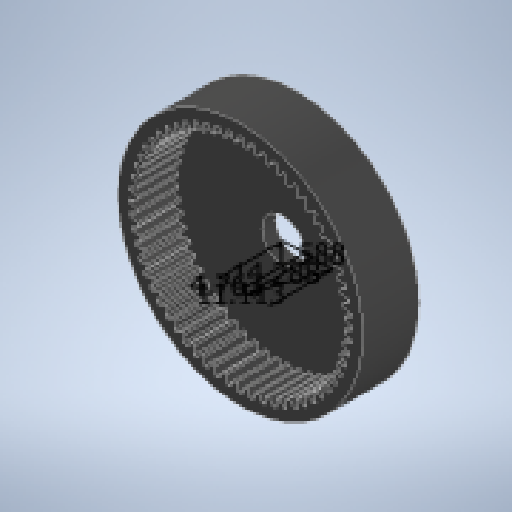
# Autodesk Inventor part: Spur Gear2
Saved by Autodesk Inventor 2023.2 (Build 272271000, 271)
## iProperties
CustomPartVersion: 1
Created: 2023-02-28
Part Number: Spur Gear2
Material: Nylon 6/6
Document SubType Name: Modeling
Designer: Nathan Cai
Categories: <?xml version="1.0" encoding="UTF-16"?> <MemberInstance><Categories><FamilyTemplate><FamilyTemplateParameter ValueType="xs:double" Id="1" ObjectReferenceKey="da_z" ObjectType="kUserParameterObject"/><FamilyTemplateParameter ValueType="xs:double" Id="2" ObjectReferenceKey="da_b" ObjectType="kUserParameterObject"/><FamilyTemplateParameter ValueType="xs:double" Id="3" ObjectReferenceKey="da_beta" ObjectType="kUserParameterObject"/><FamilyTemplateParameter ValueType="xs:double" Id="4" ObjectReferenceKey="da_da" ObjectType="kUserParameterObject"/><FamilyTemplateParameter ValueType="xs:double" Id="5" ObjectReferenceKey="da_aw" ObjectType="kUserParameterObject"/><FamilyTemplateParameter ValueType="xs:string" Id="6" ObjectReferenceKey="EAIAABAAAACIAQAAAAAAAIAAAAAAAAAA" ObjectType="83910656" SubObjectId="SurfaceGeometry"/></FamilyTemplate><ParamToTemplateMap><ParamToTemplate CategoryParameter="//CategoryParameter[@InternalName='046C89C9-8512-4d59-83FE-43B91F4F132A']" TemplateParameter="1"/><ParamToTemplate CategoryParameter="//CategoryParameter[@InternalName='2552DF32-E462-4b46-AEBF-C6C7768E72AC']" TemplateParameter="2"/><ParamToTemplate CategoryParameter="//CategoryParameter[@InternalName='C9EE641D-15FC-4fae-A226-E94C4372FDD7']" TemplateParameter="3"/><ParamToTemplate><ParamToTemplate CategoryParameter="//CategoryParameter[@InternalName='00B6519A-459B-49c7-AD84-2E56D39A5744']" ConstantValue="-0.000000"/></ParamToTemplate><ParamToTemplate><ParamToTemplate CategoryParameter="//CategoryParameter[@InternalName='04B31F0E-C7A6-4894-AA32-9629BEFACF47']" ConstantValue="1.000000"/></ParamToTemplate><ParamToTemplate><ParamToTemplate CategoryParameter="//CategoryParameter[@InternalName='43CBEC2E-7847-49e7-A936-2F7889FCB2D9']" ConstantValue="0.250000"/></ParamToTemplate><ParamToTemplate><ParamToTemplate CategoryParameter="//CategoryParameter[@InternalName='B1EFC894-105D-4ebd-86BF-FA20ED196853']" ConstantValue="0.350000"/></ParamToTemplate><ParamToTemplate><ParamToTemplate CategoryParameter="//CategoryParameter[@InternalName='51175063-3D10-4879-93E8-6246FE8B403D']" ConstantValue="2060000000.000000"/></ParamToTemplate><ParamToTemplate><ParamToTemplate CategoryParameter="//CategoryParameter[@InternalName='A3A52E27-4454-46a9-B0BD-C932399B70AF']" ConstantValue="0.300000"/></ParamToTemplate><ParamToTemplate><ParamToTemplate CategoryParameter="//CategoryParameter[@InternalName='91B76062-C214-41d9-B1B9-14D2AB99603D']" ConstantValue="0.080000"/></ParamToTemplate><ParamToTemplate><ParamToTemplate CategoryParameter="//CategoryParameter[@InternalName='374E806E-8B8A-4dda-A9AA-1039D6500AD2']" ConstantValue="12.500000"/></ParamToTemplate><ParamToTemplate><ParamToTemplate CategoryParameter="//CategoryParameter[@InternalName='2D373A89-B862-43d6-8D0B-0CBF12AB9F6C']" ConstantValue="0.349066"/></ParamToTemplate><ParamToTemplate CategoryParameter="//CategoryParameter[@InternalName='37777632-D6A2-4fac-9D53-DB8ACD95C989']" TemplateParameter="4"/><ParamToTemplate CategoryParameter="//CategoryParameter[@InternalName='FD1017F1-B727-4f7e-9707-0F86F1FF9423']" TemplateParameter="5"/><ParamToTemplate><ParamToTemplate CategoryParameter="//CategoryParameter[@InternalName='9E1B4470-B2D3-4ff1-B813-535BB4CDF51A']" ConstantValue="3520000.000000"/></ParamToTemplate><ParamToTemplate><ParamToTemplate CategoryParameter="//CategoryParameter[@InternalName='F8452263-BFF6-458c-9FB1-07C4B99E95CD']" ConstantValue="11400000.000000"/></ParamToTemplate><ParamToTemplate><ParamToTemplate CategoryParameter="//CategoryParameter[@InternalName='3E3BB259-FD49-497f-8171-6EBC954A3479']" ConstantValue="2.000000"/></ParamToTemplate><ParamToTemplate CategoryParameter="//CategoryParameter[@InternalName='27C3BAF2-7550-4e4b-AE2C-0DB134B7D9B7']" TemplateParameter="6"/></ParamToTemplateMap><Category DisplayName="Gear" InternalName="DC85795E-93AB-48d5-8EEE-5A27447B64BD" Mnemonic="Gear"><CategoryParameter DisplayName="z" InternalName="046C89C9-8512-4d59-83FE-43B91F4F132A" Mnemonic="z"/><CategoryParameter DisplayName="b" InternalName="2552DF32-E462-4b46-AEBF-C6C7768E72AC" Mnemonic="b"/><CategoryParameter DisplayName="||b|" InternalName="C9EE641D-15FC-4fae-A226-E94C4372FDD7" Mnemonic="beta"/><CategoryParameter DisplayName="x" InternalName="00B6519A-459B-49c7-AD84-2E56D39A5744" Mnemonic="x"/><CategoryParameter DisplayName="a*" InternalName="04B31F0E-C7A6-4894-AA32-9629BEFACF47" Mnemonic="a"/><CategoryParameter DisplayName="c*" InternalName="43CBEC2E-7847-49e7-A936-2F7889FCB2D9" Mnemonic="c"/><CategoryParameter DisplayName="r|.f|*" InternalName="B1EFC894-105D-4ebd-86BF-FA20ED196853" Mnemonic="rf"/><CategoryParameter DisplayName="E" InternalName="51175063-3D10-4879-93E8-6246FE8B403D" Mnemonic="E"/><CategoryParameter DisplayName="||m|" InternalName="A3A52E27-4454-46a9-B0BD-C932399B70AF" Mnemonic="mi"/><Category DisplayName="SpurGear" InternalName="26C5A22E-A91E-4dfd-A3B3-23CCAFAE1764" Mnemonic="SpurGear"><CategoryParameter DisplayName="m" InternalName="91B76062-C214-41d9-B1B9-14D2AB99603D" Mnemonic="m"/><CategoryParameter DisplayName="P" InternalName="374E806E-8B8A-4dda-A9AA-1039D6500AD2" Mnemonic="PP"/><CategoryParameter DisplayName="||a|" InternalName="2D373A89-B862-43d6-8D0B-0CBF12AB9F6C" Mnemonic="alpha"/><CategoryParameter DisplayName="d|.a|" InternalName="37777632-D6A2-4fac-9D53-DB8ACD95C989" Mnemonic="da"/><CategoryParameter DisplayName="a|.w|" InternalName="FD1017F1-B727-4f7e-9707-0F86F1FF9423" Mnemonic="aw"/><CategoryParameter DisplayName="||s||.Flim|" InternalName="9E1B4470-B2D3-4ff1-B813-535BB4CDF51A" Mnemonic="sFlim"/><CategoryParameter DisplayName="||s||.Hlim|" InternalName="F8452263-BFF6-458c-9FB1-07C4B99E95CD" Mnemonic="sHlim"/><CategoryParameter DisplayName="type" InternalName="3E3BB259-FD49-497f-8171-6EBC954A3479" Mnemonic="type"/><Category DisplayName="InternalSpurGear" InternalName="7CF704F6-14A9-42f8-93CE-E71DF57C2B55" Mnemonic="InternalSpurGear"><CategoryParameter DisplayName="PitchDiameter" InternalName="27C3BAF2-7550-4e4b-AE2C-0DB134B7D9B7" Mnemonic="IDS_PITCHDIAM"/></Category></Category></Category></Categories></MemberInstance>
Density: 1.13 g/cm^3
Appearance: Rubber - Black
Mass: 12.9636 g
Surface Area: 87.0105 cm^2
Volume: 11.4722 cm^3
Author: Nathan Cai
Autodesk Inventor part; units mm, degrees
ref_plane "YZ Plane" through (0, 0, 0) normal (1, 0, 0) x (0, 1, 0)
ref_plane "XZ Plane" through (0, 0, 0) normal (0, 1, 0) x (-1, 0, 0)
ref_plane "XY Plane" through (0, 0, 0) normal (0, 0, 1) x (1, 0, 0)
sketch "Sketch1" plane through (0, 0, 0) normal (0, 0, 1) x (1, 0, 0)
  circle A0 centre (0, 0) radius 27.5
  dimension "d0" = 55
  constraints: 1 centre point
  measures "d0" diameter of A0
extrude "Extrusion1" add sketch "Sketch1" along normal blind 9.525
spur gear teeth "Spur Gear" teeth 60 pitch diameter 48 tip diameter 46.7556 root diameter 50 face width 9.525 start plane through (0, 0, 0) normal (0, 0, -1) x (-1, 0, 0)
sketch "Sketch4" plane through (0, 0, 0) normal (0, 0, -1) x (-1, 0, 0)
  circle A0 centre (0, 0) radius 27.5
  circle A1 centre (0, 0) radius 4.7625
  dimension "d55" = 55
  dimension "d56" = 9.525
  constraints: 2 centre point, 2 coincident
  measures "d55" diameter of A0
  measures "d56" diameter of A1
extrude "Extrusion2" add sketch "Sketch4" along normal blind 3.175 from surface at 0
sketch "Sketch10" plane through (0, 0, -3.175) normal (0, 0, -1) x (-1, 0, 0)
  circle A0 centre (0, 0) radius 4.7625
  circle A1 centre (0, 0) radius 7.1438
  dimension "d83" = 9.525
  dimension "d84" = 14.2875
  constraints: 2 centre point, 2 coincident
  measures "d83" diameter of A0
  measures "d84" diameter of A1
extrude "Extrusion6" add sketch "Sketch10" against normal blind 17.4625
chamfer "Chamfer1" distance 3.175 distance2 14.2875 1 edges at (7.1438, 0, 0) measured on face at (7.6438, 0, 0)
sketch "Sketch15" plane through (0, 0, -3.175) normal (0, 0, -1) x (-1, 0, 0)
  circle A0 centre (0, 0) radius 33.3375
  dimension "d109" = 66.675
  constraints: 1 centre point, 1 coincident
  measures "d109" diameter of A0
extrude "Extrusion9" add sketch "Sketch15" against normal blind 3.175
chamfer "Chamfer2" distance 3.175 angle 45 1 edges at (-27.5, 0, 0)
sketch "Sketch13" plane through (0, 0, -3.175) normal (0, 0, -1) x (-1, 0, 0)
  circle A0 centre (0, 0) radius 27.5
  circle A1 centre (0, 0) radius 38.1 construction
  circle A2 centre (0, 0) radius 33.3375
  line L0 (-1.5875, -35) -> (1.5875, -35)
  line L1 (1.5875, -35) -> (1.5875, 35)
  line L2 (1.5875, 35) -> (-1.5875, 35)
  line L3 (-1.5875, 35) -> (-1.5875, -35)
  line L4 (-1.5875, -35) -> (1.5875, 35) construction
  line L5 (1.5875, -35) -> (-1.5875, 35) construction
  circle A3 centre (0, 0) radius 30.9563
  line L6 (0, 0) -> (5.789, 32.831)
  line L7 (0, 0) -> (0, 33.3375) construction
  line L8 (0, 0) -> (-5.789, 32.831)
  line L9 (0, 0) -> (-21.4289, 25.538)
  line L10 (-18.8748, 29.5171) -> (16.1252, -31.1046)
  line L11 (18.8748, -29.5171) -> (-16.1252, 31.1046)
  line L12 (0, 0) -> (-11.4021, 31.327)
  line L13 (0, 0) -> (-31.327, 11.4021)
  line L14 (-31.1046, 16.1252) -> (29.5171, -18.8748)
  line L15 (31.1046, -16.1252) -> (-29.5171, 18.8748)
  line L16 (0, 0) -> (-25.538, 21.4289)
  line L17 (0, 0) -> (-32.831, -5.789)
  line L18 (-35, -1.5875) -> (35, -1.5875)
  line L19 (35, 1.5875) -> (-35, 1.5875)
  line L20 (0, 0) -> (-32.831, 5.789)
  line L21 (0, 0) -> (-25.538, -21.4289)
  line L22 (-29.5171, -18.8748) -> (31.1046, 16.1252)
  line L23 (29.5171, 18.8748) -> (-31.1046, -16.1252)
  line L24 (0, 0) -> (-31.327, -11.4021)
  line L25 (0, 0) -> (-11.4021, -31.327)
  line L26 (-16.1252, -31.1046) -> (18.8748, 29.5171)
  line L27 (16.1252, 31.1046) -> (-18.8748, -29.5171)
  line L28 (0, 0) -> (-21.4289, -25.538)
  line L29 (0, 0) -> (5.789, -32.831)
  line L30 (1.5875, -35) -> (1.5875, 35)
  line L31 (-1.5875, 35) -> (-1.5875, -35)
  line L32 (0, 0) -> (-5.789, -32.831)
  line L33 (0, 0) -> (21.4289, -25.538)
  line L34 (18.8748, -29.5171) -> (-16.1252, 31.1046)
  line L35 (-18.8748, 29.5171) -> (16.1252, -31.1046)
  line L36 (0, 0) -> (11.4021, -31.327)
  line L37 (0, 0) -> (31.327, -11.4021)
  line L38 (31.1046, -16.1252) -> (-29.5171, 18.8748)
  line L39 (-31.1046, 16.1252) -> (29.5171, -18.8748)
  line L40 (0, 0) -> (25.538, -21.4289)
  line L41 (0, 0) -> (32.831, 5.789)
  line L42 (35, 1.5875) -> (-35, 1.5875)
  line L43 (-35, -1.5875) -> (35, -1.5875)
  line L44 (0, 0) -> (32.831, -5.789)
  line L45 (0, 0) -> (25.538, 21.4289)
  line L46 (29.5171, 18.8748) -> (-31.1046, -16.1252)
  line L47 (-29.5171, -18.8748) -> (31.1046, 16.1252)
  line L48 (0, 0) -> (31.327, 11.4021)
  line L49 (0, 0) -> (11.4021, 31.327)
  line L50 (16.1252, 31.1046) -> (-18.8748, -29.5171)
  line L51 (-16.1252, -31.1046) -> (18.8748, 29.5171)
  line L52 (0, 0) -> (21.4289, 25.538)
  point P0 (5.3755, 30.486)
  point P1 (-5.3755, 30.486)
  point P2 (-1.5875, 30.9155)
  point P3 (-1.5875, 27.4541)
  point P4 (1.5875, 27.4541)
  point P5 (1.5875, 30.9155)
  point P6 (-23.7139, 19.8983)
  point P7 (-29.0894, 10.5877)
  point P8 (-27.5674, 14.0829)
  point P9 (-24.5697, 12.3523)
  point P10 (-22.9822, 15.1019)
  point P11 (-25.9799, 16.8326)
  point P12 (-30.486, 5.3755)
  point P13 (-30.486, -5.3755)
  point P14 (-30.9155, -1.5875)
  point P15 (-27.4541, -1.5875)
  point P16 (-27.4541, 1.5875)
  point P17 (-30.9155, 1.5875)
  point P18 (-23.7139, -19.8983)
  point P19 (-25.9799, -16.8326)
  point P20 (-22.9822, -15.1019)
  point P21 (-24.5697, -12.3523)
  point P22 (-27.5674, -14.0829)
  point P23 (-29.0894, -10.5877)
  point P24 (-15.1019, -22.9822)
  point P25 (-16.8326, -25.9799)
  point P26 (-19.8983, -23.7139)
  point P27 (-10.5877, -29.0894)
  point P28 (-14.0829, -27.5674)
  point P29 (-12.3523, -24.5697)
  point P30 (1.5875, -30.9155)
  point P31 (1.5875, -27.4541)
  point P32 (-1.5875, -27.4541)
  point P33 (-1.5875, -30.9155)
  point P34 (-5.3755, -30.486)
  point P35 (5.3755, -30.486)
  point P36 (16.8326, -25.9799)
  point P37 (15.1019, -22.9822)
  point P38 (12.3523, -24.5697)
  point P39 (14.0829, -27.5674)
  point P40 (10.5877, -29.0894)
  point P41 (19.8983, -23.7139)
  point P42 (29.0894, -10.5877)
  point P43 (27.5674, -14.0829)
  point P44 (24.5697, -12.3523)
  point P45 (22.9822, -15.1019)
  point P46 (25.9799, -16.8326)
  point P47 (23.7139, -19.8983)
  point P48 (30.486, 5.3755)
  point P49 (30.9155, 1.5875)
  point P50 (27.4541, 1.5875)
  point P51 (27.4541, -1.5875)
  point P52 (30.9155, -1.5875)
  point P53 (30.486, -5.3755)
  point P54 (25.9799, 16.8326)
  point P55 (22.9822, 15.1019)
  point P56 (24.5697, 12.3523)
  point P57 (27.5674, 14.0829)
  point P58 (29.0894, 10.5877)
  point P59 (23.7139, 19.8983)
  point P60 (10.5877, 29.0894)
  point P61 (14.0829, 27.5674)
  point P62 (12.3523, 24.5697)
  point P63 (15.1019, 22.9822)
  point P64 (16.8326, 25.9799)
  point P65 (19.8983, 23.7139)
  point P66 (-10.5877, 29.0894)
  point P67 (-19.8983, 23.7139)
  point P68 (-16.8326, 25.9799)
  point P69 (-15.1019, 22.9822)
  point P70 (-12.3523, 24.5697)
  point P71 (-14.0829, 27.5674)
  dimension "d92" = 55
  dimension "d97" = 2.3813
  dimension "d93" = 76.2
  dimension "d94" = 4.7625
  dimension "d95" = 3.175
  dimension "d96" = 70
  dimension "d98" = 10
  dimension "d101" = 360
  constraints: 106 end point, 4 coincident, 2 midpoint, 2 parallel, 1 centre point, 1 horizontal, 1 perpendicular, 1 symmetric about line, 1 vertical, 141 other
  measures "d93" diameter of A1
  measures "d95" distance of L2.end L1.end
  measures "d96" distance of L1.end L0.end
  measures "d98" angle of L7 L6
extrude "Extrusion7" add sketch "Sketch13" against normal blind 12.7 contours A0 L19 A3 L18 | L19 A2 L18 A3 | A3 L41 A2 L19 | L18 A2 L44 A3 | A0 L23 A3 L22 | A3 L22 A2 L48 | L15 A3 L14 A0 | L37 A2 L15 A3 | A3 L23 A2 L22 | L15 A2 L14 A3 | A3 L45 A2 L23 | L14 A2 L40 A3 | A0 L27 A3 L26 | A3 L26 A2 L52 | L11 A3 L10 A0 | L33 A2 L11 A3 | A3 L27 A2 L26 | L11 A2 L10 A3 | A3 L49 A2 L27 | L10 A2 L36 A3 | A0 L3 A3 L1 | A3 L1 A2 L6 | L1 A3 L3 A0 | L29 A2 L1 A3 | A3 L3 A2 L1 | L1 A2 L3 A3 | A3 L8 A2 L3 | L3 A2 L32 A3 | L10 A3 L11 A0 | L14 A3 L15 A0 | L18 A3 L19 A0 | L22 A3 L23 A0 | L26 A3 L27 A0 | A3 L11 A2 L12 | L9 A2 L10 A3 | L10 A2 L11 A3 | L13 A2 L14 A3 | L14 A2 L15 A3 | L15 A2 L16 A3 | L17 A2 L18 A3 | L18 A2 L19 A3 | L19 A2 L20 A3 | L21 A2 L22 A3 | L22 A2 L23 A3 | L23 A2 L24 A3 | L25 A2 L26 A3 | L26 A2 L27 A3 | L27 A2 L28 A3
equation "\"d0\" = 1.1 * da_df"
equation "\"d1\" = da_b"
equation "\"d16\" = da_aw"
equation "\"d47\" = da_aw"
equation "\"d52\" = da_aw"
equation "\"da_df\" = 50"
equation "\"da_b\" = 9.525"
equation "\"da_aw\" = 18"
body "Solid1"
